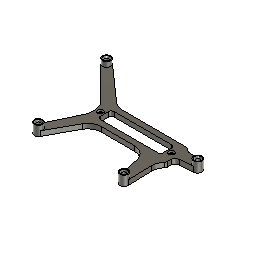
SKR_E3_DIN_mount (Autodesk Fusion 360 design; units mm, degrees)
Autodesk Fusion 360 part; units mm, degrees
sketch "Sketch1" plane through (0, 0, 0) normal (0, 0, 1) x (1, 0, 0)
  circle A0 centre (-53.3684, 32.1159) radius 1.4
  circle A1 centre (-53.3684, 32.1159) radius 3
  circle A2 centre (42.3116, 2.3474) radius 3.05
  circle A3 centre (42.3116, 2.3474) radius 1.4
  circle A4 centre (-38.1495, -32.3541) radius 3.05
  circle A5 centre (-38.1495, -32.3541) radius 1.4
  circle A6 centre (24.0005, -32.6326) radius 3.05
  circle A7 centre (24.0005, -32.6326) radius 1.4
  line L0 (-28.8453, -0.7789) -> (-28.8407, -3.1456)
  line L1 (29.7254, -6.7498) -> (29.7402, -4.3316)
  arc A8 (29.4751, 7.9011) -> (27.8129, 8.7977) centre (27.8058, 6.7953) ccw
  line L2 (-18.9251, 8.9631) -> (27.8129, 8.7977)
  circle A9 centre (25.5857, 0.0088) radius 1.2
  line L3 (22.6857, 2.9886) -> (22.6857, -2.9886)
  line L4 (-20.8143, 4.9886) -> (20.6857, 4.9886)
  circle A10 centre (25.65, 0) radius 1.2
  line L5 (7.8719, -9.0318) -> (-15.9654, -9.0153)
  arc A11 (22.6857, 2.9886) -> (20.6857, 4.9886) centre (20.6857, 2.9886) ccw
  line L6 (20.6857, -4.9886) -> (-20.8143, -4.9886)
  arc A12 (29.2124, -8.4036) -> (29.7254, -6.7498) centre (27.7423, -7.0411) ccw
  arc A13 (-20.8143, 4.9886) -> (-22.8143, 2.9886) centre (-20.8143, 2.9886) ccw
  arc A14 (-22.8143, -2.9886) -> (-20.8143, -4.9886) centre (-20.8143, -2.9886) ccw
  circle A15 centre (-25.7143, 0.0088) radius 1.2
  line L7 (-22.8143, -2.9886) -> (-22.8143, 2.9886)
  arc A16 (20.6857, -4.9886) -> (22.6857, -2.9886) centre (20.6857, -2.9886) ccw
  line L8 (-51.3802, 34.3625) -> (-25.5169, 11.4744)
  line L9 (42.6416, 5.3795) -> (31.6517, 6.5753)
  line L10 (42.5132, -0.696) -> (32.5418, -1.3565)
  line L11 (-55.49, 29.9949) -> (-31.7733, 6.2718)
  line L12 (-35.4741, -33.8184) -> (-24.7444, -14.2142)
  line L13 (-40.9094, -31.0559) -> (-29.7918, -7.4216)
  line L14 (21.0135, -33.2497) -> (17.6582, -17.0085)
  line L15 (27.0492, -32.5436) -> (26.5512, -15.4928)
  arc A17 (-25.5169, 11.4744) -> (-18.9251, 8.9631) centre (-18.8897, 18.9631) ccw
  arc A18 (-28.8453, -0.7789) -> (-31.7733, 6.2718) centre (-38.8453, -0.7983) ccw
  arc A19 (-29.7918, -7.4216) -> (-28.8407, -3.1456) centre (-38.8407, -3.165) ccw
  arc A20 (-15.9654, -9.0153) -> (-24.7444, -14.2142) centre (-15.9723, -19.0153) ccw
  arc A21 (17.6582, -17.0085) -> (7.8719, -9.0318) centre (7.865, -19.0317) ccw
  arc A22 (29.2124, -8.4036) -> (26.5512, -15.4928) centre (36.547, -15.2009) ccw
  arc A23 (32.5418, -1.3565) -> (29.7402, -4.3316) centre (32.7401, -4.3499) ccw
  arc A24 (29.4751, 7.9011) -> (31.6517, 6.5753) centre (31.9762, 9.5577) ccw
  circle A25 centre (-25.7143, 0.0088) radius 2
  circle A26 centre (25.65, 0) radius 2
  dimension "d1" = 1.6
  dimension "d3" = 1.6
  dimension "d4" = 1.6
  dimension "d5" = 1.6
  dimension "d8" = 2.8
  dimension "d9" = 6.1
  dimension "d10" = 2.8
  dimension "d11" = 6.1
  dimension "d12" = 2.8
  dimension "d13" = 6.1
  dimension "d14" = 2.8
  dimension "d17" = 2
  dimension "d18" = 10
  dimension "d19" = 3
  dimension "d20" = 62.15
  dimension "d21" = 34.98
  dimension "d22" = 95.68
  dimension "d23" = 64.47
  dimension "d24" = 3.5
  dimension "d25" = 3.5
  dimension "d26" = 10
  dimension "d27" = 10
  dimension "d30" = 0.8
  dimension "d31" = 0.8
  dimension "d44" = 45.5
  dimension "d45" = 51.3
  dimension "d46" = 2.9
  dimension "d47" = 2.9
  constraint tangent A8 L2
  constraint tangent L1 A8
  constraint tangent L5 A12
  constraint horizontal L6
  constraint perpendicular L6 L7
  constraint parallel L4 L6
  constraint parallel L3 L7
  constraint tangent A13 L7
  constraint tangent L4 A13
  constraint tangent L6 A14
  constraint tangent A14 L7
  constraint equal A13 A14
  constraint tangent L6 A16
  constraint tangent L3 A16
  constraint equal A13 A16
  constraint tangent L3 A11
  constraint tangent L4 A11
  constraint equal A11 A13
  constraint coincident A2 L9.start
  constraint coincident A2 L10.start
  constraint tangent A2 L10
  constraint tangent A2 L9
  constraint coincident A1 L11.start
  constraint tangent A1 L11
  constraint tangent L8 A17
  constraint tangent L2 A17
  constraint tangent L11 A18
  constraint tangent L0 A18
  constraint equal A17 A18
  constraint tangent L13 A19
  constraint tangent L0 A19
  constraint equal A17 A19
  constraint tangent L12 A20
  constraint tangent L5 A20
  constraint equal A17 A20
  constraint tangent L14 A21
  constraint tangent L5 A21
  constraint equal A17 A21
  constraint tangent L15 A22
  constraint tangent A12 A22
  constraint equal A17 A22
  constraint tangent L10 A23
  constraint tangent L1 A23
  constraint tangent L9 A24
  constraint tangent A8 A24
  constraint equal A23 A24
  constraint coincident A1 L8.start
  constraint coincident A6 L15.start
  constraint coincident A6 L14.start
  constraint coincident A4 L13.start
  constraint tangent A4 L13
  constraint coincident A4 L12.start
  constraint tangent A4 L12
  constraint tangent A6 L15
  constraint tangent A6 L14
  constraint tangent A1 L8
  measures "d8" diameter of A7
  measures "d9" diameter of A6
  measures "d10" diameter of A5
  measures "d11" diameter of A4
  measures "d12" diameter of A3
  measures "d13" diameter of A2
  measures "d14" diameter of A0
  measures "d17" radius of A13
  measures "d18" radius of A17
  measures "d19" radius of A23
  measures "d20" horizontal distance of A4.centre A6.centre
  measures "d21" vertical distance of A2.centre A6.centre
  measures "d22" horizontal distance of A0.centre A2.centre
  measures "d23" vertical distance of A0.centre A4.centre
  measures "d24" angle of L12 L13
  measures "d25" angle of L8 L11
  measures "d26" angle of L9 L10
  measures "d27" angle of L14 L15
  measures "d44" distance of L3 L7
  measures "d45" distance of A15.centre A9.centre
  measures "d46" distance of A9.centre L3
  measures "d47" distance of A15.centre L7
extrude "Extrude1" add sketch "Sketch1" against normal blind 3.5 contours A1 | A1 A2 A4 A6 L0 L1 A8 L2 L5 A12 L8 L9 L10 L11 L12 L13 L14 L15 A17 A18 A19 A20 A21 A22 A23 A24 | A4 | A2 | A6 | A25 | A26
extrude "Extrude2" cut sketch "Sketch1" against normal blind 1.5 contours A25 | A26
extrude "Extrude3" add sketch "Sketch1" along normal blind 3.5 contours A1 | A4 | A2 | A6
chamfer "Chamfer1" distance 1 angle 45 4 edges at (22.6952, -32.1264, 3.5) (41.0064, 2.8536, 3.5) (-54.6736, 32.6222, 3.5) (-39.4548, -31.8478, 3.5)
chamfer "Chamfer2" distance 0.5 angle 45 3 edges at (26.8388, -0.1634, -3.5) (24.3968, 0.1723, -3.5) (-26.8331, -0.4252, -3.5)
equation "d10 = d8"
equation "d11 = d9"
equation "d12 = d8"
equation "d13 = d9"
equation "d14 = d8"
equation "d46 = d47"
named bodies: "SKR E3 Mount"
